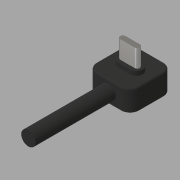
# Autodesk Inventor part: USB C Right Angle Plug
Saved by Autodesk Inventor 2019 (Build 230136000, 136)
## iProperties
Created: 2019-02-12
Part Number: USB C Right Angle Plug
Material: Generic
Document SubType Name: Modeling
Designer: Ben
Density: 1 g/cm^3
Appearance: Default
Author: Ben
Autodesk Inventor part; units mm, degrees
ref_plane "YZ Plane" through (0, 0, 0) normal (1, 0, 0) x (0, 1, 0)
ref_plane "XZ Plane" through (0, 0, 0) normal (0, 1, 0) x (-1, 0, 0)
ref_plane "XY Plane" through (0, 0, 0) normal (0, 0, 1) x (1, 0, 0)
sketch "Sketch1" plane through (0, 0, 0) normal (0, 1, 0) x (-1, 0, 0)
  line L0 (-9, 9) -> (9, 9)
  line L1 (9, 9) -> (9, -9)
  line L2 (9, -9) -> (-9, -9)
  line L3 (-9, -9) -> (-9, 9)
  line L4 (-9, 9) -> (9, -9) construction
  line L5 (9, 9) -> (-9, -9) construction
  point P0 (0, 0)
  dimension "d0" = 18
  dimension "d1" = 18
  constraints: 12 end point, 2 midpoint, 2 parallel, 1 horizontal, 1 perpendicular
  measures "d0" distance of L1.end L2.end
  measures "d1" distance of L0.end L1.end
extrude "Extrusion1" add sketch "Sketch1" along normal blind 9
fillet "Fillet1" radius 0.75 8 edges at (0, 9, 9) (9, 9, 0) (0, 9, -9) (-9, 9, 0) (0, 0, 9) (-9, 0, 0) (0, 0, -9) (9, 0, 0)
fillet "Fillet2" radius 4 12 edges at (-8.7803, 8.7803, 8.7803) (-8.7803, 0.2197, 8.7803) (-9, 4.5, 9) (8.7803, 8.7803, 8.7803) (8.7803, 0.2197, 8.7803) (9, 4.5, 9) (8.7803, 8.7803, -8.7803) (8.7803, 0.2197, -8.7803) (9, 4.5, -9) (-8.7803, 8.7803, -8.7803) (-8.7803, 0.2197, -8.7803) (-9, 4.5, -9)
sketch "Sketch2" plane through (0, 9, 0) normal (0, 1, 0) x (1, 0, 0)
  line L0 (0, 0) -> (-5.25, 0) construction
  line L1 (-5.25, 0) -> (5.25, 0) construction
  line L2 (-2.625, -2.625) -> (2.625, -2.625)
  line L3 (2.625, 2.625) -> (-2.625, 2.625)
  arc A0 (-2.625, 2.625) -> (-2.625, -2.625) centre (-2.625, 0) ccw
  arc A1 (2.625, -2.625) -> (2.625, 2.625) centre (2.625, 0) ccw
  dimension "d6" = 5.25
  dimension "d7" = 10.5
  dimension "d8" = 5.25
  constraints: 10 end point, 6 point on circle, 4 tangent, 3 point on line, 2 centre point, 1 horizontal, 1 midpoint, 1 parallel
  measures "d6" distance of L0.start L0.end
  measures "d7" distance of L0.end L1.end
  measures "d8" diameter of A1
extrude "Extrusion2" add sketch "Sketch2" along normal blind 1.75
sketch "Sketch3" plane through (0, 10.75, 0) normal (0, 1, 0) x (1, 0, 0)
  line L0 (0, 0) -> (-4.125, 0) construction
  line L1 (-4.125, 0) -> (4.125, 0) construction
  line L2 (-3, -1.125) -> (3, -1.125)
  line L3 (3, 1.125) -> (-3, 1.125)
  arc A0 (-3, 1.125) -> (-3, -1.125) centre (-3, 0) ccw
  arc A1 (3, -1.125) -> (3, 1.125) centre (3, 0) ccw
  dimension "d11" = 4.125
  dimension "d12" = 8.25
  dimension "d13" = 2.25
  constraints: 10 end point, 6 point on circle, 4 tangent, 3 point on line, 2 centre point, 1 horizontal, 1 midpoint, 1 parallel
  measures "d11" distance of L0.start L0.end
  measures "d12" distance of L0.end L1.end
  measures "d13" diameter of A1
extrude "Extrusion3" add sketch "Sketch3" along normal blind 7.45 separate body
sketch "Sketch4" plane through (-5, 8.25, 9) normal (0, 0, 1) x (1, 0, 0)
  line L0 (10, 0) -> (10, -7.5) construction
  line L1 (0, 0) -> (10, 0) construction
  line L2 (0, -7.5) -> (0, 0) construction
  line L3 (10, -7.5) -> (0, -7.5) construction
  line L4 (10, -7.5) -> (0, -7.5) construction
  line L5 (5, -7.5) -> (5, 0) construction
  circle A0 centre (5, -3.75) radius 3
  point P0 (5, -8.25)
  dimension "d16" = 6
  constraints: 3 midpoint, 2 end point, 1 centre point
  measures "d16" diameter of A0
extrude "Extrusion4" add sketch "Sketch4" along normal blind 33.5 bodies 1
equation "\"d7\" = 2 * d6"
equation "\"d8\" = d6"
body "Solid1"
body "Solid2"
